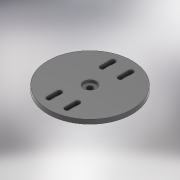
# Autodesk Inventor part: BaseGear
Saved by Autodesk Inventor 2020.3 (Build 243373000, 373)
## iProperties
Created: 2021-08-03
Part Number: BaseGear
Material: ABS Plastic
Document SubType Name: Modeling
Designer: justi
Density: 1.06 g/cm^3
Appearance: Smooth - Black
Author: justi
Autodesk Inventor part; units mm, degrees
ref_plane "YZ Plane" through (0, 0, 0) normal (1, 0, 0) x (0, 1, 0)
ref_plane "XZ Plane" through (0, 0, 0) normal (0, 1, 0) x (-1, 0, 0)
ref_plane "XY Plane" through (0, 0, 0) normal (0, 0, 1) x (1, 0, 0)
sketch "Sketch1" plane through (0, 0, 0) normal (0, 1, 0) x (-1, 0, 0)
  circle A0 centre (0, 0) radius 48
  dimension "d0" = 96
  constraints: 1 centre point, 1 coincident
  measures "d0" diameter of A0
extrude "Extrusion1" add sketch "Sketch1" along normal blind 5
sketch "Sketch2" plane through (0, 5, 0) normal (0, 1, 0) x (1, 0, 0)
  line L0 (13, -30.5) -> (13, 30.5) construction
  line L1 (13, 30.5) -> (-13, 30.5) construction
  line L2 (-13, 30.5) -> (-13, -30.5) construction
  line L3 (-13, -30.5) -> (13, -30.5) construction
  line L4 (13, -30.5) -> (-13, 30.5) construction
  line L5 (13, 30.5) -> (-13, -30.5) construction
  line L6 (-13, -30.5) -> (-10.25, -30.5)
  line L7 (-13, 30.5) -> (-10.25, 30.5)
  line L8 (13, -30.5) -> (10.25, -30.5) construction
  line L9 (13, 30.5) -> (10.25, 30.5)
  line L10 (10.25, -36.5) -> (10.25, -24.5) construction
  line L11 (13, -36.5) -> (13, -24.5)
  line L12 (7.5, -24.5) -> (7.5, -36.5)
  arc A0 (7.5, -36.5) -> (13, -36.5) centre (10.25, -36.5) ccw
  arc A1 (13, -24.5) -> (7.5, -24.5) centre (10.25, -24.5) ccw
  line L13 (-7.5, -36.5) -> (-7.5, -24.5)
  line L14 (-13, -24.5) -> (-13, -36.5)
  arc A2 (-13, -36.5) -> (-7.5, -36.5) centre (-10.25, -36.5) ccw
  arc A3 (-7.5, -24.5) -> (-13, -24.5) centre (-10.25, -24.5) ccw
  line L15 (13, 24.5) -> (13, 36.5)
  line L16 (7.5, 36.5) -> (7.5, 24.5)
  arc A4 (7.5, 24.5) -> (13, 24.5) centre (10.25, 24.5) ccw
  arc A5 (13, 36.5) -> (7.5, 36.5) centre (10.25, 36.5) ccw
  line L17 (-7.5, 24.5) -> (-7.5, 36.5)
  line L18 (-13, 36.5) -> (-13, 24.5)
  arc A6 (-13, 24.5) -> (-7.5, 24.5) centre (-10.25, 24.5) ccw
  arc A7 (-7.5, 36.5) -> (-13, 36.5) centre (-10.25, 36.5) ccw
  point P0 (0, 0)
  point P1 (0, 0)
  dimension "d3" = 61
  dimension "d4" = 26
  dimension "d5" = 2.75
  dimension "d6" = 2.75
  dimension "d7" = 2.75
  dimension "d8" = 2.75
  dimension "d9" = 6
  dimension "d10" = 5.5
  dimension "d11" = 6
  dimension "d12" = 5.5
  dimension "d13" = 6
  dimension "d14" = 5.5
  dimension "d15" = 6
  dimension "d16" = 5.5
  constraints: 40 end point, 16 point on circle, 16 tangent, 8 centre point, 6 parallel, 4 point on line, 3 midpoint, 2 vertical, 1 coincident, 1 perpendicular
  measures "d3" distance of L0.start L0.end
  measures "d4" distance of L1.end L0.end
  measures "d5" distance of L2.end L6.end
  measures "d6" distance of L1.end L7.end
  measures "d7" distance of L0.start L8.end
  measures "d8" distance of L0.end L9.end
  measures "d9" distance of L8.end L10.end
  measures "d10" diameter of A1
  measures "d11" distance of point (-10.25, -30.5) A3.centre
  measures "d12" diameter of A3
  measures "d13" distance of point (10.25, 30.5) A5.centre
  measures "d14" diameter of A5
  measures "d15" distance of point (-10.25, 30.5) A7.centre
  measures "d16" diameter of A7
extrude "Extrusion2" cut sketch "Sketch2" against normal through all
sketch "Sketch3" plane through (0, 0, 0) normal (0, -1, 0) x (1, 0, 0)
  circle A0 centre (0, 0) radius 7.275
  line L0 (7.275, 0) -> (-7.275, 0) construction
  line L1 (0, 7.275) -> (0, -7.275) construction
  line L2 (9.775, 2.5) -> (4.775, 2.5)
  line L3 (4.775, 2.5) -> (4.775, -2.5)
  line L4 (4.775, -2.5) -> (9.775, -2.5)
  line L5 (9.775, -2.5) -> (9.775, 2.5)
  line L6 (9.775, 2.5) -> (4.775, -2.5) construction
  line L7 (4.775, 2.5) -> (9.775, -2.5) construction
  line L8 (2.5, 9.775) -> (-2.5, 9.775)
  line L9 (-2.5, 9.775) -> (-2.5, 4.775)
  line L10 (-2.5, 4.775) -> (2.5, 4.775)
  line L11 (2.5, 4.775) -> (2.5, 9.775)
  line L12 (2.5, 9.775) -> (-2.5, 4.775) construction
  line L13 (-2.5, 9.775) -> (2.5, 4.775) construction
  line L14 (-9.775, 2.5) -> (-4.775, 2.5)
  line L15 (-4.775, 2.5) -> (-4.775, -2.5)
  line L16 (-4.775, -2.5) -> (-9.775, -2.5)
  line L17 (-9.775, -2.5) -> (-9.775, 2.5)
  line L18 (-9.775, 2.5) -> (-4.775, -2.5) construction
  line L19 (-4.775, 2.5) -> (-9.775, -2.5) construction
  line L20 (-2.5, -4.775) -> (2.5, -4.775)
  line L21 (2.5, -4.775) -> (2.5, -9.775)
  line L22 (2.5, -9.775) -> (-2.5, -9.775)
  line L23 (-2.5, -9.775) -> (-2.5, -4.775)
  line L24 (-2.5, -4.775) -> (2.5, -9.775) construction
  line L25 (2.5, -4.775) -> (-2.5, -9.775) construction
  point P0 (6.832, 2.5)
  point P1 (2.5, 6.832)
  point P2 (-2.5, 6.832)
  point P3 (-6.832, 2.5)
  point P4 (-6.832, -2.5)
  point P5 (-2.5, -6.832)
  point P6 (2.5, -6.832)
  point P7 (6.832, -2.5)
  dimension "d20" = 14.55
  dimension "d21" = 5
  dimension "d22" = 5
  dimension "d23" = 5
  dimension "d24" = 5
  dimension "d25" = 5
  dimension "d26" = 5
  dimension "d27" = 5
  dimension "d28" = 5
  constraints: 52 end point, 8 midpoint, 8 parallel, 5 horizontal, 5 perpendicular, 4 point on circle, 1 centre point, 1 coincident
  measures "d20" diameter of A0
  measures "d21" distance of L4.end L3.end
  measures "d22" distance of L3.end L2.end
  measures "d23" distance of L10.end L9.end
  measures "d24" distance of L9.end L8.end
  measures "d25" distance of L15.end L16.end
  measures "d26" distance of L14.end L15.end
  measures "d27" distance of L21.end L22.end
  measures "d28" distance of L20.end L21.end
extrude "Extrusion3" add sketch "Sketch3" along normal blind 5 contours L2 L3 L4 A0 L21 L20 L23 L16 L15 L14 L9 L10 L11
hole "Hole1" at (0, 5, 0) direction (0, -1, 0) diameter 6.6 end through all counterbore diameter 14.55 counterbore depth 3 clearance for "Hex Head Bolt" size "M6" standard "Ansi Metric M Profile"
body "Solid1"
